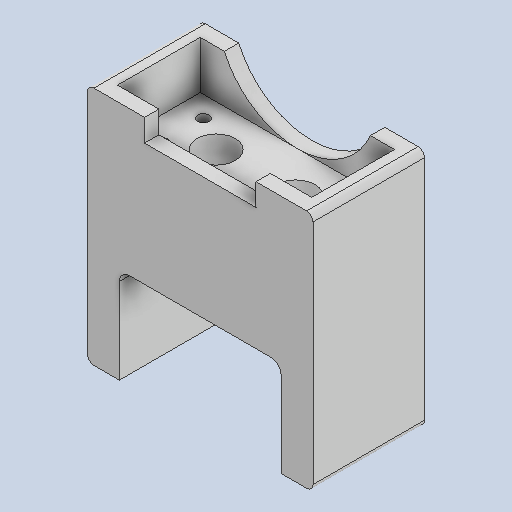
# Autodesk Inventor part: BK12_Spacer
Saved by Autodesk Inventor 2023 (Build 270158000, 158)
## iProperties
Created: 2022-05-04
Part Number: BK12_Spacer
Material: Generic
Document SubType Name: Modeling
Designer: plebbb
Density: 1 g/cm^3
Appearance: Default
Mass: 101.961 g
Surface Area: 235.547 cm^2
Volume: 101.961 cm^3
Author: plebbb
Autodesk Inventor part; units mm, degrees
ref_plane "YZ Plane" through (0, 0, 0) normal (1, 0, 0) x (0, 1, 0)
ref_plane "XZ Plane" through (0, 0, 0) normal (0, 1, 0) x (-1, 0, 0)
ref_plane "XY Plane" through (0, 0, 0) normal (0, 0, 1) x (1, 0, 0)
sketch "Sketch1" plane through (0, 0, 0) normal (0, 1, 0) x (-1, 0, 0)
  line L0 (0, 0) -> (60, 0) construction
  line L1 (60, 0) -> (60, -25) construction
  line L2 (60, -25) -> (0, -25) construction
  line L3 (0, -25) -> (0, 0) construction
  line L4 (60.5, 0.5) -> (-0.5, 0.5)
  line L5 (-0.5, 0.5) -> (-0.5, -25.5)
  line L6 (-0.5, -25.5) -> (60.5, -25.5)
  line L7 (60.5, -25.5) -> (60.5, 0.5)
  circle A0 centre (53, -19) radius 1.8
  circle A1 centre (7, -19) radius 1.8
  circle A2 centre (7, -6) radius 1.8
  circle A3 centre (53, -6) radius 1.8
  line L8 (53, -19) -> (7, -19) construction
  line L9 (7, -19) -> (7, -6) construction
  point P0 (30, -19)
  point P1 (30, -25)
  point P2 (7, -12.5)
  point P3 (0, -12.5)
  dimension "d0" = 25
  dimension "d1" = 60
  dimension "d2" = 0.5
  dimension "d3" = 0.5
  dimension "d4" = 0.5
  dimension "d5" = 0.5
  dimension "d6" = 3.6
  dimension "d7" = 46
  dimension "d8" = 13
  constraints: 20 end point, 4 centre point, 4 midpoint, 4 parallel, 3 equal radius, 3 horizontal, 3 horizontal alignment, 3 perpendicular, 3 vertical alignment
  measures "d0" distance of L0.end L1.end
  measures "d1" distance of L1.end L2.end
  measures "d2" distance between parallel lines of L7 L1
  measures "d3" distance between parallel lines of L5 L3
  measures "d4" distance between parallel lines of L6 L2
  measures "d5" distance between parallel lines of L4 L0
  measures "d6" diameter of A0
  measures "d7" distance of L8.start L8.end
  measures "d8" distance of L8.end L9.end
sketch "Sketch2" plane through (0, 0, 0) normal (0, 1, 0) x (-1, 0, 0)
  line L0 (-5.4, 5) -> (65.4, 5)
  line L1 (65.4, 5) -> (65.4, -30)
  line L2 (65.4, -30) -> (-5.4, -30)
  line L3 (-5.4, -30) -> (-5.4, 5)
  line L4 (60.5, -25.5) -> (60.5, 0.5) construction
  line L5 (-0.5, 0.5) -> (-0.5, -25.5) construction
  line L6 (-0.5, -25.5) -> (60.5, -25.5) construction
  point P0 (0, 0)
  point P1 (60.5, -12.5)
  point P2 (65.4, -12.5)
  point P3 (30, -25.5)
  point P4 (30, -30)
  dimension "d9" = 70.8
  dimension "d10" = 35
  constraints: 8 end point, 4 midpoint, 2 parallel, 1 horizontal, 1 horizontal alignment, 1 perpendicular, 1 vertical alignment
  measures "d9" distance of L1.end L2.end
  measures "d10" distance of L0.end L1.end
extrude "Extrusion1" add sketch "Sketch2" along normal blind 10 and the other way blind 35.4
extrude "Extrusion2" cut sketch "Sketch1" along normal blind 10 and the other way blind 5
extrude "Extrusion3" cut sketch "Sketch1" along normal blind 10 and the other way blind 30.4 contours A0 | A1 | A2 | A3
sketch "Sketch3" plane through (5.4, 10, -30) normal (0, 0, -1) x (-1, 0, 0)
  line L0 (70.8, -45.4) -> (0, -45.4) projected
  line L1 (0, -45.4) -> (0, -75.4)
  line L2 (0, -75.4) -> (10, -75.4)
  line L3 (10, -75.4) -> (10, -48.575)
  line L4 (13.175, -45.4) -> (57.625, -45.4)
  line L5 (60.8, -48.575) -> (60.8, -75.4)
  line L6 (60.8, -75.4) -> (70.8, -75.4)
  line L7 (70.8, -75.4) -> (70.8, -45.4)
  arc A0 (13.175, -45.4) -> (10, -48.575) centre (13.175, -48.575) ccw
  arc A1 (60.8, -48.575) -> (57.625, -45.4) centre (57.625, -48.575) ccw
  point P0 (5.4, -10)
  point P1 (10, -45.4)
  point P2 (60.8, -45.4)
  point P3 (35.4, -45.4)
  point P4 (13.175, -45.4)
  point P5 (57.625, -45.4)
  dimension "d23" = 50.8
  dimension "d24" = 3.175
  dimension "d25" = 10
  dimension "d26" = 30
  constraints: 14 end point, 6 point on line, 5 perpendicular, 4 point on circle, 4 tangent, 2 centre point, 2 midpoint, 1 equal radius, 1 vertical
  measures "d23" distance of point (10, -45.4) point (60.8, -45.4)
  measures "d24" radius of A0
  measures "d25" distance of L1.end L2.end
  measures "d26" distance of L0.end L1.end
extrude "Extrusion4" add sketch "Sketch3" against normal up to surface (35 mm away)
sketch "Sketch4" plane through (0, -5, 0) normal (0, 1, 0) x (1, 0, 0)
  circle A0 centre (-42.5, 12.5) radius 3
  circle A1 centre (-17.5, 12.5) radius 3
  line L0 (-60.5, 25.5) -> (0.5, 25.5) construction
  line L1 (-60.5, -0.5) -> (-60.5, 25.5) construction
  line L2 (-42.5, 12.5) -> (-17.5, 12.5) construction
  point P0 (0, 0)
  point P1 (-30, 25.5)
  point P2 (-30, 12.5)
  point P3 (-60.5, 12.5)
  dimension "d29" = 6
  dimension "d30" = 25
  constraints: 3 midpoint, 2 centre point, 2 end point, 1 equal radius, 1 horizontal, 1 horizontal alignment, 1 vertical alignment
  measures "d29" diameter of A0
  measures "d30" distance of L2.start L2.end
extrude "Extrusion5" cut sketch "Sketch4" against normal up to surface (30.4 mm away)
sketch "Sketch5" plane through (0, -5, 0) normal (0, 1, 0) x (1, 0, 0)
  circle A0 centre (-42.5, 12.5) radius 3 construction
  circle A1 centre (-17.5, 12.5) radius 3 construction
  circle A2 centre (-17.5, 12.5) radius 6
  circle A3 centre (-42.5, 12.5) radius 6
  point P0 (0, 0)
  dimension "d34" = 12
  constraints: 2 centre point, 2 concentric, 1 equal radius
  measures "d34" diameter of A3
extrude "Extrusion6" cut sketch "Sketch5" against normal blind 10
fillet "Fillet1" radius 2 2 edges at (-65.4, 10, -12.5) (5.4, 10, -12.5)
fillet "Fillet2" radius 2 2 edges at (-65.4, -65.4, -12.5) (5.4, -65.4, -12.5)
sketch "Sketch6" plane through (-52.225, -35.4, 5) normal (0, 0, 1) x (1, 0, 0)
  line L0 (44.45, 0) -> (0, 0) construction
  line L1 (4.725, 38.4) -> (39.725, 38.4)
  line L2 (44.45, 0) -> (0, 0) projected
  line L3 (-11.175, 45.4) -> (55.625, 45.4) projected
  line L4 (39.725, 38.4) -> (39.725, 45.4)
  line L5 (4.725, 38.4) -> (4.725, 45.4)
  point P0 (52.225, 35.4)
  point P1 (22.225, 38.4)
  point P2 (22.225, 0)
  point P3 (70.325, 0)
  point P4 (-0.475, 0)
  dimension "d39" = 38.4
  dimension "d40" = 35
  constraints: 8 end point, 2 midpoint, 2 perpendicular, 2 point on line, 1 horizontal, 1 vertical alignment
  measures "d39" distance between parallel lines of L0 L1
  measures "d40" distance of L1.start L1.end
extrude "Extrusion7" cut sketch "Sketch6" against normal up to surface (4.5 mm away)
sketch "Sketch7" plane through (-4.6, -65.4, -30) normal (0, 0, -1) x (-1, 0, 0)
  arc A0 (2.4871, 75.4) -> (48.3129, 75.4) centre (25.4, 85.4) ccw
  line L0 (-8, 75.4) -> (58.8, 75.4) projected
  point P0 (-4.6, 65.4)
  point P1 (25.4, 75.4)
  dimension "d44" = 25
  dimension "d45" = 10
  constraints: 2 point on circle, 2 point on line, 1 centre point, 1 midpoint, 1 vertical alignment
  measures "d44" radius of A0
  measures "d45" distance from line of L0 A0.centre
extrude "Extrusion8" cut sketch "Sketch7" against normal blind 10
body "Solid1"
